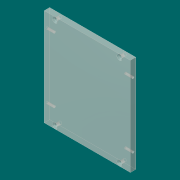
# Autodesk Inventor part: front
Saved by Autodesk Inventor 2016 (Build 200138000, 138)
## iProperties
Created: 2015-10-13
Part Number: front
Material: PC/ABS Plastic
Document SubType Name: Modeling
Designer: Sawaiz
Density: 0.357273 g/cm^3
Appearance: Clear
Author: Sawaiz
Autodesk Inventor part; units mm, degrees
ref_plane "YZ Plane" through (0, 0, 0) normal (1, 0, 0) x (0, 1, 0)
ref_plane "XZ Plane" through (0, 0, 0) normal (0, 1, 0) x (-1, 0, 0)
ref_plane "XY Plane" through (0, 0, 0) normal (0, 0, 1) x (1, 0, 0)
sketch "Sketch1" plane through (0, 0, 0) normal (1, 0, 0) x (0, 1, 0)
  line L0 (-50, -56.35) -> (50, -56.35)
  line L1 (50, -56.35) -> (50, 56.35)
  line L2 (50, 56.35) -> (-50, 56.35)
  line L3 (-50, 56.35) -> (-50, -56.35)
  line L4 (-50, -56.35) -> (50, 56.35) construction
  line L5 (50, -56.35) -> (-50, 56.35) construction
  point P0 (0, 0)
  dimension "d0" = 100
  dimension "d1" = 112.7
  constraints: 12 end point, 2 midpoint, 2 parallel, 1 horizontal, 1 perpendicular
  measures "d0" distance of L2.end L1.end
  measures "d1" distance of L1.end L0.end
extrude "Extrusion1" add sketch "Sketch1" along normal blind 6.35
sketch "Sketch2" plane through (6.35, 0, 0) normal (1, 0, 0) x (0, 0, -1)
  line L0 (56.35, -50) -> (56.35, 50) projected
  line L1 (56.35, 50) -> (-56.35, 50) projected
  line L2 (-56.35, 50) -> (-56.35, -50) projected
  line L3 (-56.35, -50) -> (56.35, -50) projected
  line L4 (-53.175, -50) -> (-53.175, 50)
  point P0 (0, 0)
  point P1 (-53.175, -37.5)
  point P2 (-53.175, -12.5)
  point P3 (-53.175, 12.5)
  point P4 (-53.175, 37.5)
  dimension "d4" = 3.175
  dimension "d5" = 12.5
  dimension "d6" = 12.5
  dimension "d7" = 25
  dimension "d8" = 25
  constraints: 6 point on line, 2 end point, 1 vertical
  measures "d4" distance between parallel lines of L2 L4
  measures "d5" vertical distance of point (0, 0) point (-53.175, 12.5)
  measures "d6" vertical distance of point (0, 0) point (-53.175, -12.5)
  measures "d7" distance of point (-53.175, -12.5) point (-53.175, -37.5)
  measures "d8" distance of point (-53.175, 37.5) point (-53.175, 12.5)
hole "Hole1" at (6.35, -37.5, 53.175) at (6.35, 37.5, 53.175) direction (-1, 0, 0) diameter 3.4 end through all countersink diameter 6.3 countersink angle 90 clearance for "Flat Head Machine Screw" size "M3" standard "Ansi Metric M Profile"
mirror "Mirror1" about plane through (0, 0, 0) normal (0, 0, 1) of "Hole1"
sketch "Sketch3" plane through (0, 50, 56.35) normal (0, 1, 0) x (1, 0, 0)
  line L0 (0, 112.7) -> (0, 0) projected
  line L1 (0, 0) -> (6.35, 0) projected
  line L2 (6.35, 112.7) -> (6.35, 0) projected
  line L3 (0, 112.7) -> (6.35, 112.7) projected
  line L4 (3.175, 0) -> (3.175, 112.7)
  point P0 (0, 56.35)
  point P1 (3.175, 18.85)
  point P2 (3.175, 43.85)
  point P3 (3.175, 68.85)
  point P4 (3.175, 93.85)
  dimension "d16" = 12.5
  dimension "d17" = 12.5
  dimension "d18" = 25
  dimension "d19" = 25
  constraints: 4 point on line, 2 end point, 2 midpoint
  measures "d16" vertical distance of point (0, 56.35) point (3.175, 43.85)
  measures "d17" vertical distance of point (0, 56.35) point (3.175, 68.85)
  measures "d18" distance of point (3.175, 43.85) point (3.175, 18.85)
  measures "d19" distance of point (3.175, 68.85) point (3.175, 93.85)
hole "Hole2" at (3.175, 50, 37.5) at (3.175, 50, -37.5) direction (0, -1, 0) diameter 2.459 depth 8.8 tip angle 118 thread size "M3x0.5" class "6H" standard "ANSI Metric M Profile"
mirror "Mirror2" about plane through (0, 0, 0) normal (0, 1, 0) of "Hole2"
equation "\"d0\" = width"
equation "\"d1\" = height + 2 * acrylicThickness"
equation "\"d2\" = acrylicThickness"
equation "\"d4\" = 0.5 * acrylicThickness"
equation "\"d5\" = 0.125 * width"
equation "\"d6\" = 0.125 * width"
equation "\"d7\" = 0.25 * width"
equation "\"d8\" = 0.25 * width"
equation "\"d16\" = 0.125 * height"
equation "\"d17\" = 0.125 * height"
equation "\"d18\" = 0.25 * height"
equation "\"d19\" = 0.25 * height"
equation "\"acrylicThickness\" = 6.35"
equation "\"width\" = 100"
equation "\"mirrorAngle\" = 17deg"
equation "\"detectorWidth\" = 52"
equation "\"detectorHeight\" = 52"
equation "\"mirrorThickness\" = 3"
equation "\"fresnelThickness\" = 0.1"
equation "\"ior\" = 1.49"
equation "\"focalLength\" = 76.2"
equation "\"fresnelAngle\" = 90deg"
equation "\"centerThickness\" = 1.524"
equation "\"fresnelEffectiveDiameter\" = 76.2"
equation "\"height\" = 100"
body "Solid1"
